Autodesk Fusion 360 part; units mm, degrees
(part 3 of 3)
extrude "Extruir4" cut sketch "Boceto5" against normal blind 3 contours S7 L81 L82 L83 L84 L85 L86 L87 L88 L89 L90 L91 L92 S8 L93 L94 L95 L96 L97 L98 L99 L100 L101 L102 L103 L104 L105 L106 L107 L108 L109 L110 L111 L112 L113 L114 L115 L116 L117 L118 L119 L120 L121 L122 L123 L124 S9 S10 L125 L126 | S15 L179 L180 S16 L181 L182 L183 L184 L185 L186 L187 L188 L189 L190 L191 L192 L193 L194 L195 L196 S17 L197 L198 L199 L200 L201 L202 L203 L204 S18 S19 L205 L206 L207 L208 S20 L209 L210 L211 L212 L213 L214 S21 L215 L216 L217 L218 S22 L219 L220 L221 L222 | L269 L270 S29 L271 L272 L273 L274 L275 L276 L277 L278 L279 L280 S30 L281 L282 S31 L283 L284 S32 L285 L286 L287 L288 L289 L290 L291 L292 L293 L294 L295 L296 L297 L298 L299 L300 L301 L302 L303 L304 L305 L306 L307 L308 S33 L309 L310 L311 L312 | L363 L364 S41 L365 L366 S42 L367 L368 L369 L370 L371 L372 S43 L373 L374 L375 L376 S44 L377 L378 L379 L380 L381 L382 L383 L384 S45 L385 L386 L387 L388 L389 L390 L391 L392 S46 L393 L394 L395 L396 L397 L398 L399 L400 L401 L402 L403 L404 L405 L406 L407 L408 L409 L410 | L451 L452 L453 L454 L455 L456 S57 L457 L458 L459 L460 L461 L462 L463 L464 L465 L466 S58 S59 S60 L467 L468 L469 L470 L471 L472 L473 L474 S61 L475 L476 L477 L478 L479 L480 L481 L482 L483 L484 L485 L486 L487 L488 S62 S63 S64 L489 L490 L491 L492 S65 | L541 L542 S70 L543 L544 L545 L546 L547 L548 L549 L550 L551 L552 L553 L554 L555 L556 S71 L557 L558 L559 L560 L561 L562 L563 L564 L565 L566 L567 L568 L569 L570 S72 L571 L572 L573 L574 L575 L576 L577 L578 L579 L580 L581 L582 L583 L584 S73 L585 L586 L587 L588 | L627 L628 L629 L630 L631 L632 L633 L634 L635 L636 L637 L638 L639 L640 L641 L642 L643 L644 L645 L646 L647 L648 L649 L650 L651 L652 L653 L654 L655 L656 L657 L658 L659 L660 L661 L662 L663 L664 L665 L666 L667 L668 L669 L670 L671 L672 L673 L674 L675 L676 S81 L677 L678 L679 L680 L681 L682 | S89 L723 L724 L725 L726 L727 L728 S90 L729 L730 L731 L732 L733 L734 S91 S92 S93 L735 L736 L737 L738 L739 L740 L741 L742 L743 L744 L745 L746 L747 L748 L749 L750 L751 L752 L753 L754 L755 L756 L757 L758 S94 S95 L759 L760 L761 L762 L763 L764 L765 L766 | S102 L815 L816 L817 L818 S103 L819 L820 L821 L822 L823 L824 L825 L826 L827 L828 L829 L830 L831 L832 L833 L834 L835 L836 S104 L837 L838 L839 L840 S105 L841 L842 S106 L843 L844 S107 L845 L846 L847 L848 L849 L850 S108 L851 L852 L853 L854 S109 L855 L856 | L903 L904 S117 L905 L906 S118 L907 L908 L909 L910 L911 L912 L913 L914 L915 L916 S119 L917 L918 L919 L920 L921 L922 L923 L924 L925 L926 L927 L928 L929 L930 L931 L932 L933 L934 S120 L935 L936 L937 L938 L939 L940 S121 L941 L942 L943 L944 | L985 L986 S129 S130 L987 L988 L989 L990 L991 L992 L993 L994 L995 L996 L997 L998 L999 L1000 L1001 L1002 S131 L1003 L1004 L1005 L1006 L1007 L1008 L1009 L1010 S132 L1011 L1012 L1013 L1014 L1015 L1016 L1017 L1018 L1019 L1020 L1021 L1022 S133 L1023 L1024 L1025 L1026 L1027 L1028 L1029 L1030 L1031 L1032 L1033 L1034 | S141 L1079 L1080 L1081 L1082 L1083 L1084 L1085 L1086 L1087 L1088 L1089 L1090 L1091 L1092 L1093 L1094 S142 L1095 L1096 L1097 L1098 S143 L1099 L1100 L1101 L1102 L1103 L1104 L1105 L1106 L1107 L1108 L1109 L1110 S144 L1111 L1112 L1113 L1114 S145 L1115 L1116 L1117 L1118 S146 L1119 L1120 L1121 L1122 L1123 L1124 L1125 L1126 bodies 2
sketch "Boceto7" plane through (0, -37, 0) normal (0, 1, 0) x (-1, 0, 0)
  line L0 (14.5856, 106.9791) -> (14.4281, 107.0187)
  line L1 (14.4281, 107.0187) -> (14.3014, 107.078)
  spline S0 degree 3 poles (14.3014, 107.078) (14.2318, 107.1106) (11.7179, 108.5531) (8.7151, 110.2835) knots 0 0 0 0 1 1 1 1
  line L2 (8.7151, 110.2835) -> (3.2554, 113.4298)
  line L3 (3.2554, 113.4298) -> (3.1368, 113.5206)
  spline S1 degree 3 poles (3.1368, 113.5206) (3.0715, 113.5705) (2.9644, 113.6706) (2.8986, 113.743) knots 0 0 0 0 1 1 1 1
  line L4 (2.8986, 113.743) -> (2.7791, 113.8747)
  line L5 (2.7791, 113.8747) -> (2.6095, 114.1591)
  line L6 (2.6095, 114.1591) -> (2.5502, 114.3319)
  line L7 (2.5502, 114.3319) -> (2.4909, 114.5047)
  line L8 (2.4909, 114.5047) -> (2.469, 114.6412)
  spline S2 degree 3 poles (2.469, 114.6412) (2.4006, 115.0677) (2.504, 115.4998) (2.7672, 115.888) knots 0 0 0 0 1 1 1 1
  line L9 (2.7672, 115.888) -> (2.8507, 116.0112)
  line L10 (2.8507, 116.0112) -> (2.9755, 116.136)
  line L11 (2.9755, 116.136) -> (3.1003, 116.2607)
  line L12 (3.1003, 116.2607) -> (3.2424, 116.3527)
  spline S3 degree 3 poles (3.2424, 116.3527) (3.3206, 116.4033) (3.4405, 116.4695) (3.509, 116.4999) knots 0 0 0 0 1 1 1 1
  line L13 (3.509, 116.4999) -> (3.6334, 116.5552)
  line L14 (3.6334, 116.5552) -> (3.9904, 116.6432)
  line L15 (3.9904, 116.6432) -> (4.2109, 116.6419)
  line L16 (4.2109, 116.6419) -> (4.4315, 116.6407)
  line L17 (4.4315, 116.6407) -> (4.5995, 116.5962)
  line L18 (4.5995, 116.5962) -> (4.7675, 116.5517)
  line L19 (4.7675, 116.5517) -> (4.9145, 116.4817)
  spline S4 degree 3 poles (4.9145, 116.4817) (5.0975, 116.3946) (15.7827, 110.2419) (15.9754, 110.1127) knots 0 0 0 0 1 1 1 1
  line L20 (15.9754, 110.1127) -> (16.1156, 110.0186)
  line L21 (16.1156, 110.0186) -> (16.2617, 109.8648)
  line L22 (16.2617, 109.8648) -> (16.4079, 109.7109)
  line L23 (16.4079, 109.7109) -> (16.497, 109.561)
  line L24 (16.497, 109.561) -> (16.586, 109.4111)
  line L25 (16.586, 109.4111) -> (16.7046, 109.0654)
  line L26 (16.7046, 109.0654) -> (16.7265, 108.9289)
  spline S5 degree 3 poles (16.7265, 108.9289) (16.7385, 108.8538) (16.7485, 108.7329) (16.7486, 108.6602) knots 0 0 0 0 1 1 1 1
  line L27 (16.7486, 108.6602) -> (16.7487, 108.5281)
  line L28 (16.7487, 108.5281) -> (16.7154, 108.3662)
  line L29 (16.7154, 108.3662) -> (16.682, 108.2044)
  line L30 (16.682, 108.2044) -> (16.6212, 108.0463)
  line L31 (16.6212, 108.0463) -> (16.5603, 107.8883)
  line L32 (16.5603, 107.8883) -> (16.4558, 107.7291)
  line L33 (16.4558, 107.7291) -> (16.3513, 107.5699)
  line L34 (16.3513, 107.5699) -> (16.1738, 107.4019)
  line L35 (16.1738, 107.4019) -> (15.9964, 107.234)
  line L36 (15.9964, 107.234) -> (15.6251, 107.0427)
  line L37 (15.6251, 107.0427) -> (15.4744, 106.9972)
  line L38 (15.4744, 106.9972) -> (15.3236, 106.9516)
  line L39 (15.3236, 106.9516) -> (15.1804, 106.9351)
  line L40 (15.1804, 106.9351) -> (15.0371, 106.9187)
  line L41 (15.0371, 106.9187) -> (14.8901, 106.9291)
  line L42 (14.8901, 106.9291) -> (14.7431, 106.9395)
  line L43 (14.7431, 106.9395) -> (14.5856, 106.9791)
  line L44 (-15.008, 106.9658) -> (-15.1472, 106.9935)
  line L45 (-15.1472, 106.9935) -> (-15.3104, 107.0614)
  line L46 (-15.3104, 107.0614) -> (-15.4735, 107.1293)
  line L47 (-15.4735, 107.1293) -> (-15.6249, 107.2305)
  line L48 (-15.6249, 107.2305) -> (-15.7763, 107.3318)
  line L49 (-15.7763, 107.3318) -> (-15.9106, 107.4743)
  spline S6 degree 3 poles (-15.9106, 107.4743) (-15.9844, 107.5526) (-16.0816, 107.6722) (-16.1266, 107.7401) knots 0 0 0 0 1 1 1 1
  line L50 (-16.1266, 107.7401) -> (-16.2083, 107.8634)
  line L51 (-16.2083, 107.8634) -> (-16.278, 108.0344)
  line L52 (-16.278, 108.0344) -> (-16.3477, 108.2054)
  line L53 (-16.3477, 108.2054) -> (-16.3823, 108.4044)
  line L54 (-16.3823, 108.4044) -> (-16.4168, 108.6034)
  line L55 (-16.4168, 108.6034) -> (-16.4028, 108.7786)
  line L56 (-16.4028, 108.7786) -> (-16.3888, 108.9539)
  line L57 (-16.3888, 108.9539) -> (-16.3374, 109.1312)
  line L58 (-16.3374, 109.1312) -> (-16.2861, 109.3085)
  line L59 (-16.2861, 109.3085) -> (-16.2151, 109.4495)
  spline S7 degree 3 poles (-16.2151, 109.4495) (-16.086, 109.7058) (-15.8768, 109.9466) (-15.6462, 110.1044) knots 0 0 0 0 1 1 1 1
  spline S8 degree 3 poles (-15.6462, 110.1044) (-15.4992, 110.205) (-4.6465, 116.4518) (-4.5256, 116.5054) knots 0 0 0 0 1 1 1 1
  spline S9 degree 3 poles (-4.5256, 116.5054) (-4.4621, 116.5336) (-4.3392, 116.5755) (-4.2526, 116.5985) knots 0 0 0 0 1 1 1 1
  line L60 (-4.2526, 116.5985) -> (-4.0951, 116.6404)
  line L61 (-4.0951, 116.6404) -> (-3.6121, 116.6404)
  line L62 (-3.6121, 116.6404) -> (-3.2783, 116.552)
  line L63 (-3.2783, 116.552) -> (-3.1092, 116.47)
  line L64 (-3.1092, 116.47) -> (-2.94, 116.3879)
  line L65 (-2.94, 116.3879) -> (-2.8017, 116.2831)
  spline S10 degree 3 poles (-2.8017, 116.2831) (-2.6357, 116.1572) (-2.5152, 116.0251) (-2.3869, 115.8283) knots 0 0 0 0 1 1 1 1
  line L66 (-2.3869, 115.8283) -> (-2.2913, 115.6818)
  line L67 (-2.2913, 115.6818) -> (-2.2308, 115.526)
  line L68 (-2.2308, 115.526) -> (-2.1703, 115.3701)
  line L69 (-2.1703, 115.3701) -> (-2.1404, 115.2138)
  line L70 (-2.1404, 115.2138) -> (-2.1105, 115.0576)
  line L71 (-2.1105, 115.0576) -> (-2.1105, 114.7235)
  line L72 (-2.1105, 114.7235) -> (-2.1437, 114.5616)
  line L73 (-2.1437, 114.5616) -> (-2.177, 114.3997)
  line L74 (-2.177, 114.3997) -> (-2.2405, 114.2466)
  line L75 (-2.2405, 114.2466) -> (-2.3041, 114.0935)
  line L76 (-2.3041, 114.0935) -> (-2.4037, 113.9421)
  line L77 (-2.4037, 113.9421) -> (-2.5034, 113.7907)
  line L78 (-2.5034, 113.7907) -> (-2.6482, 113.6524)
  spline S11 degree 3 poles (-2.6482, 113.6524) (-2.7278, 113.5763) (-2.845, 113.4803) (-2.9085, 113.4391) knots 0 0 0 0 1 1 1 1
  spline S12 degree 3 poles (-2.9085, 113.4391) (-3.069, 113.3348) (-13.7648, 107.1737) (-13.9105, 107.1015) knots 0 0 0 0 1 1 1 1
  spline S13 degree 3 poles (-13.9105, 107.1015) (-13.9755, 107.0693) (-14.0965, 107.0224) (-14.1795, 106.9973) knots 0 0 0 0 1 1 1 1
  line L79 (-14.1795, 106.9973) -> (-14.3302, 106.9516)
  line L80 (-14.3302, 106.9516) -> (-14.4735, 106.9354)
  line L81 (-14.4735, 106.9354) -> (-14.6167, 106.9192)
  line L82 (-14.6167, 106.9192) -> (-14.7427, 106.9287)
  spline S14 degree 3 poles (-14.7427, 106.9287) (-14.812, 106.9339) (-14.9314, 106.9506) (-15.008, 106.9658) knots 0 0 0 0 1 1 1 1
  line L83 (-0.2165, 120.1648) -> (-0.3912, 120.2066)
  line L84 (-0.3912, 120.2066) -> (-0.5457, 120.278)
  spline S15 degree 3 poles (-0.5457, 120.278) (-0.7389, 120.3673) (-0.8685, 120.4553) (-1.0261, 120.6045) knots 0 0 0 0 1 1 1 1
  line L85 (-1.0261, 120.6045) -> (-1.1493, 120.7211)
  line L86 (-1.1493, 120.7211) -> (-1.2389, 120.8471)
  spline S16 degree 3 poles (-1.2389, 120.8471) (-1.3602, 121.0178) (-1.4477, 121.1975) (-1.517, 121.4184) knots 0 0 0 0 1 1 1 1
  line L87 (-1.517, 121.4184) -> (-1.5749, 121.6032)
  line L88 (-1.5749, 121.6032) -> (-1.5749, 134.561)
  line L89 (-1.5749, 134.561) -> (-1.4807, 134.9143)
  line L90 (-1.4807, 134.9143) -> (-1.3974, 135.0842)
  line L91 (-1.3974, 135.0842) -> (-1.3141, 135.254)
  line L92 (-1.3141, 135.254) -> (-1.0954, 135.5423)
  line L93 (-1.0954, 135.5423) -> (-0.9572, 135.6569)
  spline S17 degree 3 poles (-0.9572, 135.6569) (-0.7085, 135.863) (-0.4228, 135.9976) (-0.1153, 136.0535) knots 0 0 0 0 1 1 1 1
  line L94 (-0.1153, 136.0535) -> (0.0422, 136.0821)
  line L95 (0.0422, 136.0821) -> (0.3152, 136.0831)
  line L96 (0.3152, 136.0831) -> (0.5147, 136.0422)
  line L97 (0.5147, 136.0422) -> (0.7142, 136.0013)
  line L98 (0.7142, 136.0013) -> (0.9242, 135.8966)
  line L99 (0.9242, 135.8966) -> (1.1342, 135.7918)
  line L100 (1.1342, 135.7918) -> (1.2665, 135.684)
  line L101 (1.2665, 135.684) -> (1.3987, 135.5761)
  line L102 (1.3987, 135.5761) -> (1.5149, 135.4361)
  line L103 (1.5149, 135.4361) -> (1.6311, 135.2961)
  line L104 (1.6311, 135.2961) -> (1.7356, 135.0832)
  line L105 (1.7356, 135.0832) -> (1.8401, 134.8704)
  line L106 (1.8401, 134.8704) -> (1.9212, 134.477)
  line L107 (1.9212, 134.477) -> (1.9216, 121.7502)
  line L108 (1.9216, 121.7502) -> (1.8994, 121.6137)
  spline S18 degree 3 poles (1.8994, 121.6137) (1.8873, 121.5386) (1.8538, 121.4063) (1.8249, 121.3197) knots 0 0 0 0 1 1 1 1
  line L109 (1.8249, 121.3197) -> (1.7725, 121.1622)
  line L110 (1.7725, 121.1622) -> (1.6845, 121.0047)
  line L111 (1.6845, 121.0047) -> (1.5964, 120.8472)
  line L112 (1.5964, 120.8472) -> (1.3968, 120.6454)
  line L113 (1.3968, 120.6454) -> (1.1973, 120.4437)
  line L114 (1.1973, 120.4437) -> (1.0515, 120.3631)
  spline S19 degree 3 poles (1.0515, 120.3631) (0.8617, 120.2581) (0.688, 120.1888) (0.5281, 120.154) knots 0 0 0 0 1 1 1 1
  line L115 (0.5281, 120.154) -> (0.3993, 120.126)
  line L116 (0.3993, 120.126) -> (0.1788, 120.1244)
  line L117 (0.1788, 120.1244) -> (-0.0417, 120.1229)
  line L118 (-0.0417, 120.1229) -> (-0.2165, 120.1648)
  spline S20 degree 3 poles (-14.9801, 128.7007) (-15.0601, 128.7176) (-15.1906, 128.7558) (-15.2699, 128.7857) knots 0 0 0 0 1 1 1 1
  line L119 (-15.2699, 128.7857) -> (-15.4143, 128.84)
  line L120 (-15.4143, 128.84) -> (-15.568, 128.9358)
  line L121 (-15.568, 128.9358) -> (-15.7218, 129.0317)
  line L122 (-15.7218, 129.0317) -> (-15.8482, 129.1487)
  line L123 (-15.8482, 129.1487) -> (-15.9746, 129.2657)
  line L124 (-15.9746, 129.2657) -> (-16.0679, 129.3965)
  line L125 (-16.0679, 129.3965) -> (-16.1612, 129.5272)
  line L126 (-16.1612, 129.5272) -> (-16.2425, 129.7025)
  line L127 (-16.2425, 129.7025) -> (-16.3237, 129.8777)
  line L128 (-16.3237, 129.8777) -> (-16.3619, 130.0247)
  line L129 (-16.3619, 130.0247) -> (-16.4001, 130.1717)
  line L130 (-16.4001, 130.1717) -> (-16.3965, 130.6757)
  line L131 (-16.3965, 130.6757) -> (-16.3412, 130.8605)
  line L132 (-16.3412, 130.8605) -> (-16.286, 131.0452)
  line L133 (-16.286, 131.0452) -> (-16.2207, 131.1755)
  spline S21 degree 3 poles (-16.2207, 131.1755) (-16.1848, 131.2471) (-16.1143, 131.3637) (-16.0641, 131.4345) knots 0 0 0 0 1 1 1 1
  line L134 (-16.0641, 131.4345) -> (-15.9729, 131.5632)
  line L135 (-15.9729, 131.5632) -> (-15.8303, 131.6939)
  line L136 (-15.8303, 131.6939) -> (-15.6878, 131.8247)
  line L137 (-15.6878, 131.8247) -> (-15.5198, 131.9239)
  spline S22 degree 3 poles (-15.5198, 131.9239) (-15.4274, 131.9784) (-12.9324, 133.421) (-9.9754, 135.1296) knots 0 0 0 0 1 1 1 1
  line L138 (-9.9754, 135.1296) -> (-4.5991, 138.2362)
  line L139 (-4.5991, 138.2362) -> (-4.1791, 138.3825)
  line L140 (-4.1791, 138.3825) -> (-3.57, 138.3832)
  line L141 (-3.57, 138.3832) -> (-3.4335, 138.3467)
  line L142 (-3.4335, 138.3467) -> (-3.297, 138.3101)
  line L143 (-3.297, 138.3101) -> (-3.0765, 138.2007)
  line L144 (-3.0765, 138.2007) -> (-2.856, 138.0912)
  line L145 (-2.856, 138.0912) -> (-2.646, 137.8802)
  line L146 (-2.646, 137.8802) -> (-2.436, 137.6691)
  line L147 (-2.436, 137.6691) -> (-2.3655, 137.549)
  spline S23 degree 3 poles (-2.3655, 137.549) (-2.2813, 137.4053) (-2.2082, 137.2289) (-2.1624, 137.0588) knots 0 0 0 0 1 1 1 1
  line L148 (-2.1624, 137.0588) -> (-2.1289, 136.9341)
  line L149 (-2.1289, 136.9341) -> (-2.1169, 136.7338)
  line L150 (-2.1169, 136.7338) -> (-2.1048, 136.5335)
  line L151 (-2.1048, 136.5335) -> (-2.1403, 136.3584)
  spline S24 degree 3 poles (-2.1403, 136.3584) (-2.1858, 136.1342) (-2.2581, 135.9423) (-2.3658, 135.7608) knots 0 0 0 0 1 1 1 1
  line L152 (-2.3658, 135.7608) -> (-2.4513, 135.6166)
  line L153 (-2.4513, 135.6166) -> (-2.5974, 135.4627)
  line L154 (-2.5974, 135.4627) -> (-2.7436, 135.3088)
  line L155 (-2.7436, 135.3088) -> (-2.8838, 135.2147)
  spline S25 degree 3 poles (-2.8838, 135.2147) (-2.9609, 135.163) (-5.4575, 133.7148) (-8.4318, 131.9965) knots 0 0 0 0 1 1 1 1
  line L156 (-8.4318, 131.9965) -> (-13.8397, 128.8724)
  line L157 (-13.8397, 128.8724) -> (-13.9972, 128.804)
  line L158 (-13.9972, 128.804) -> (-14.1547, 128.7357)
  line L159 (-14.1547, 128.7357) -> (-14.3017, 128.7046)
  line L160 (-14.3017, 128.7046) -> (-14.4487, 128.6735)
  line L161 (-14.4487, 128.6735) -> (-14.8345, 128.6701)
  line L162 (-14.8345, 128.6701) -> (-14.9801, 128.7007)
  spline S26 degree 3 poles (-4.2618, 96.0858) (-4.3304, 96.1044) (-4.4401, 96.1413) (-4.5056, 96.1677) knots 0 0 0 0 1 1 1 1
  line L163 (-4.5056, 96.1677) -> (-4.6247, 96.2158)
  line L164 (-4.6247, 96.2158) -> (-10.0722, 99.3629)
  spline S27 degree 3 poles (-10.0722, 99.3629) (-13.0684, 101.0939) (-15.5752, 102.5473) (-15.643, 102.5927) knots 0 0 0 0 1 1 1 1
  line L165 (-15.643, 102.5927) -> (-15.7662, 102.6754)
  line L166 (-15.7662, 102.6754) -> (-16.0158, 102.925)
  line L167 (-16.0158, 102.925) -> (-16.1184, 103.0821)
  line L168 (-16.1184, 103.0821) -> (-16.2209, 103.2393)
  line L169 (-16.2209, 103.2393) -> (-16.2849, 103.4052)
  line L170 (-16.2849, 103.4052) -> (-16.3489, 103.5711)
  line L171 (-16.3489, 103.5711) -> (-16.3829, 103.7666)
  line L172 (-16.3829, 103.7666) -> (-16.4168, 103.9621)
  line L173 (-16.4168, 103.9621) -> (-16.4028, 104.1373)
  line L174 (-16.4028, 104.1373) -> (-16.3888, 104.3126)
  line L175 (-16.3888, 104.3126) -> (-16.3363, 104.4943)
  line L176 (-16.3363, 104.4943) -> (-16.2839, 104.6761)
  line L177 (-16.2839, 104.6761) -> (-16.1995, 104.8328)
  line L178 (-16.1995, 104.8328) -> (-16.1152, 104.9895)
  line L179 (-16.1152, 104.9895) -> (-16.0086, 105.121)
  spline S28 degree 3 poles (-16.0086, 105.121) (-15.8856, 105.2726) (-15.7612, 105.3819) (-15.5741, 105.5029) knots 0 0 0 0 1 1 1 1
  line L180 (-15.5741, 105.5029) -> (-15.4418, 105.5883)
  line L181 (-15.4418, 105.5883) -> (-15.2773, 105.6518)
  line L182 (-15.2773, 105.6518) -> (-15.1127, 105.7153)
  line L183 (-15.1127, 105.7153) -> (-14.9172, 105.7492)
  line L184 (-14.9172, 105.7492) -> (-14.7217, 105.7832)
  line L185 (-14.7217, 105.7832) -> (-14.5465, 105.7692)
  line L186 (-14.5465, 105.7692) -> (-14.3712, 105.7552)
  line L187 (-14.3712, 105.7552) -> (-14.1932, 105.7036)
  spline S29 degree 3 poles (-14.1932, 105.7036) (-14.0953, 105.6752) (-13.9757, 105.632) (-13.9274, 105.6075) knots 0 0 0 0 1 1 1 1
  spline S30 degree 3 poles (-13.9274, 105.6075) (-13.7892, 105.5374) (-3.0607, 99.3373) (-2.9105, 99.2406) knots 0 0 0 0 1 1 1 1
  line L188 (-2.9105, 99.2406) -> (-2.776, 99.1541)
  line L189 (-2.776, 99.1541) -> (-2.6464, 99.0264)
  line L190 (-2.6464, 99.0264) -> (-2.5167, 98.8986)
  line L191 (-2.5167, 98.8986) -> (-2.432, 98.7737)
  spline S31 degree 3 poles (-2.432, 98.7737) (-2.3086, 98.5917) (-2.2438, 98.4542) (-2.1837, 98.2468) knots 0 0 0 0 1 1 1 1
  line L192 (-2.1837, 98.2468) -> (-2.1304, 98.0629)
  line L193 (-2.1304, 98.0629) -> (-2.1176, 97.8832)
  line L194 (-2.1176, 97.8832) -> (-2.1049, 97.7036)
  line L195 (-2.1049, 97.7036) -> (-2.1576, 97.3887)
  line L196 (-2.1576, 97.3887) -> (-2.2132, 97.2312)
  spline S32 degree 3 poles (-2.2132, 97.2312) (-2.2806, 97.0402) (-2.3908, 96.8417) (-2.5188, 96.6805) knots 0 0 0 0 1 1 1 1
  line L197 (-2.5188, 96.6805) -> (-2.6142, 96.5603)
  line L198 (-2.6142, 96.5603) -> (-2.7542, 96.4448)
  line L199 (-2.7542, 96.4448) -> (-2.8943, 96.3293)
  line L200 (-2.8943, 96.3293) -> (-3.0536, 96.2468)
  spline S33 degree 3 poles (-3.0536, 96.2468) (-3.2371, 96.152) (-3.3668, 96.1052) (-3.5595, 96.0642) knots 0 0 0 0 1 1 1 1
  line L201 (-3.5595, 96.0642) -> (-3.696, 96.0353)
  line L202 (-3.696, 96.0353) -> (-3.9166, 96.0436)
  line L203 (-3.9166, 96.0436) -> (-4.1371, 96.052)
  line L204 (-4.1371, 96.052) -> (-4.2618, 96.0858)
  line L205 (18.4918, 109.3246) -> (18.2923, 109.3899)
  line L206 (18.2923, 109.3899) -> (18.1589, 109.4691)
  spline S34 degree 3 poles (18.1589, 109.4691) (18.0854, 109.5126) (17.9724, 109.591) (17.9076, 109.6432) knots 0 0 0 0 1 1 1 1
  line L207 (17.9076, 109.6432) -> (17.7897, 109.7381)
  line L208 (17.7897, 109.7381) -> (17.6666, 109.8847)
  line L209 (17.6666, 109.8847) -> (17.5434, 110.0314)
  line L210 (17.5434, 110.0314) -> (17.4504, 110.2204)
  line L211 (17.4504, 110.2204) -> (17.3573, 110.4095)
  line L212 (17.3573, 110.4095) -> (17.2632, 110.7455)
  line L213 (17.2632, 110.7455) -> (17.2508, 123.4303)
  line L214 (17.2508, 123.4303) -> (17.2729, 123.6239)
  line L215 (17.2729, 123.6239) -> (17.295, 123.8175)
  line L216 (17.295, 123.8175) -> (17.3548, 123.9956)
  line L217 (17.3548, 123.9956) -> (17.4147, 124.1736)
  line L218 (17.4147, 124.1736) -> (17.5002, 124.3165)
  spline S35 degree 3 poles (17.5002, 124.3165) (17.5472, 124.3951) (17.632, 124.5138) (17.6887, 124.5803) knots 0 0 0 0 1 1 1 1
  line L219 (17.6887, 124.5803) -> (17.7918, 124.7012)
  line L220 (17.7918, 124.7012) -> (17.937, 124.8179)
  line L221 (17.937, 124.8179) -> (18.0823, 124.9345)
  line L222 (18.0823, 124.9345) -> (18.2503, 125.0161)
  line L223 (18.2503, 125.0161) -> (18.4183, 125.0977)
  line L224 (18.4183, 125.0977) -> (18.7543, 125.1929)
  line L225 (18.7543, 125.1929) -> (19.2794, 125.1926)
  line L226 (19.2794, 125.1926) -> (19.4523, 125.1441)
  line L227 (19.4523, 125.1441) -> (19.6252, 125.0955)
  line L228 (19.6252, 125.0955) -> (19.9422, 124.9334)
  line L229 (19.9422, 124.9334) -> (20.0636, 124.8399)
  spline S36 degree 3 poles (20.0636, 124.8399) (20.1304, 124.7885) (20.2391, 124.6881) (20.305, 124.6169) knots 0 0 0 0 1 1 1 1
  line L230 (20.305, 124.6169) -> (20.425, 124.4874)
  line L231 (20.425, 124.4874) -> (20.5195, 124.3263)
  line L232 (20.5195, 124.3263) -> (20.6139, 124.1653)
  line L233 (20.6139, 124.1653) -> (20.7495, 123.7663)
  line L234 (20.7495, 123.7663) -> (20.7495, 110.7035)
  line L235 (20.7495, 110.7035) -> (20.7021, 110.54)
  line L236 (20.7021, 110.54) -> (20.6547, 110.3765)
  line L237 (20.6547, 110.3765) -> (20.5725, 110.2131)
  line L238 (20.5725, 110.2131) -> (20.4904, 110.0497)
  line L239 (20.4904, 110.0497) -> (20.373, 109.9023)
  line L240 (20.373, 109.9023) -> (20.2556, 109.755)
  line L241 (20.2556, 109.755) -> (20.1245, 109.6488)
  spline S37 degree 3 poles (20.1245, 109.6488) (19.8952, 109.4632) (19.6372, 109.3357) (19.3653, 109.2738) knots 0 0 0 0 1 1 1 1
  line L242 (19.3653, 109.2738) -> (19.2374, 109.2446)
  line L243 (19.2374, 109.2446) -> (18.9643, 109.252)
  line L244 (18.9643, 109.252) -> (18.6913, 109.2594)
  line L245 (18.6913, 109.2594) -> (18.4918, 109.3246)
  spline S38 degree 3 poles (3.947, 96.0562) (3.6813, 96.1032) (3.4436, 96.2003) (3.2159, 96.3547) knots 0 0 0 0 1 1 1 1
  line L246 (3.2159, 96.3547) -> (3.0924, 96.4384)
  line L247 (3.0924, 96.4384) -> (2.8386, 96.6956)
  line L248 (2.8386, 96.6956) -> (2.7384, 96.8488)
  line L249 (2.7384, 96.8488) -> (2.6382, 97.0019)
  line L250 (2.6382, 97.0019) -> (2.5742, 97.1678)
  line L251 (2.5742, 97.1678) -> (2.5102, 97.3337)
  line L252 (2.5102, 97.3337) -> (2.4764, 97.5292)
  line L253 (2.4764, 97.5292) -> (2.4425, 97.7247)
  line L254 (2.4425, 97.7247) -> (2.4711, 98.0549)
  line L255 (2.4711, 98.0549) -> (2.5105, 98.2052)
  spline S39 degree 3 poles (2.5105, 98.2052) (2.6122, 98.5936) (2.8445, 98.9405) (3.1621, 99.1785) knots 0 0 0 0 1 1 1 1
  line L256 (3.1621, 99.1785) -> (3.2764, 99.2641)
  line L257 (3.2764, 99.2641) -> (8.7367, 102.4202)
  line L258 (8.7367, 102.4202) -> (14.1971, 105.5763)
  line L259 (14.1971, 105.5763) -> (14.5336, 105.714)
  line L260 (14.5336, 105.714) -> (14.9321, 105.7832)
  line L261 (14.9321, 105.7832) -> (15.1074, 105.7692)
  line L262 (15.1074, 105.7692) -> (15.2826, 105.7552)
  line L263 (15.2826, 105.7552) -> (15.6461, 105.6499)
  line L264 (15.6461, 105.6499) -> (15.9623, 105.4816)
  line L265 (15.9623, 105.4816) -> (16.0977, 105.3723)
  line L266 (16.0977, 105.3723) -> (16.2331, 105.2631)
  line L267 (16.2331, 105.2631) -> (16.3447, 105.1271)
  line L268 (16.3447, 105.1271) -> (16.4563, 104.9911)
  line L269 (16.4563, 104.9911) -> (16.5586, 104.7811)
  line L270 (16.5586, 104.7811) -> (16.661, 104.5711)
  line L271 (16.661, 104.5711) -> (16.6955, 104.4346)
  line L272 (16.6955, 104.4346) -> (16.73, 104.2981)
  line L273 (16.73, 104.2981) -> (16.7415, 104.0986)
  line L274 (16.7415, 104.0986) -> (16.753, 103.8991)
  line L275 (16.753, 103.8991) -> (16.7101, 103.692)
  line L276 (16.7101, 103.692) -> (16.6671, 103.485)
  line L277 (16.6671, 103.485) -> (16.5626, 103.272)
  line L278 (16.5626, 103.272) -> (16.458, 103.059)
  line L279 (16.458, 103.059) -> (16.3418, 102.919)
  line L280 (16.3418, 102.919) -> (16.2256, 102.779)
  line L281 (16.2256, 102.779) -> (15.9743, 102.576)
  line L282 (15.9743, 102.576) -> (10.5599, 99.4468)
  spline S40 degree 3 poles (10.5599, 99.4468) (7.5821, 97.7257) (5.0794, 96.283) (4.9985, 96.2406) knots 0 0 0 0 1 1 1 1
  spline S41 degree 3 poles (4.9985, 96.2406) (4.7337, 96.102) (4.502, 96.0412) (4.22, 96.0365) knots 0 0 0 0 1 1 1 1
  line L283 (4.22, 96.0365) -> (4.0716, 96.0341)
  line L284 (4.0716, 96.0341) -> (3.947, 96.0562)
  line L285 (-19.0547, 109.2861) -> (-19.2294, 109.328)
  line L286 (-19.2294, 109.328) -> (-19.3873, 109.4009)
  line L287 (-19.3873, 109.4009) -> (-19.5453, 109.4739)
  line L288 (-19.5453, 109.4739) -> (-19.6752, 109.5666)
  line L289 (-19.6752, 109.5666) -> (-19.8051, 109.6593)
  line L290 (-19.8051, 109.6593) -> (-19.9444, 109.807)
  line L291 (-19.9444, 109.807) -> (-20.0838, 109.9547)
  line L292 (-20.0838, 109.9547) -> (-20.1723, 110.1038)
  line L293 (-20.1723, 110.1038) -> (-20.2609, 110.2528)
  line L294 (-20.2609, 110.2528) -> (-20.3203, 110.4257)
  line L295 (-20.3203, 110.4257) -> (-20.3798, 110.5985)
  line L296 (-20.3798, 110.5985) -> (-20.4022, 110.7455)
  line L297 (-20.4022, 110.7455) -> (-20.4246, 110.8925)
  line L298 (-20.4246, 110.8925) -> (-20.4129, 123.7243)
  line L299 (-20.4129, 123.7243) -> (-20.3744, 123.8608)
  line L300 (-20.3744, 123.8608) -> (-20.3359, 123.9973)
  line L301 (-20.3359, 123.9973) -> (-20.1329, 124.4173)
  line L302 (-20.1329, 124.4173) -> (-20.0167, 124.5574)
  line L303 (-20.0167, 124.5574) -> (-19.9005, 124.6974)
  line L304 (-19.9005, 124.6974) -> (-19.7683, 124.8055)
  line L305 (-19.7683, 124.8055) -> (-19.636, 124.9136)
  line L306 (-19.636, 124.9136) -> (-19.216, 125.1174)
  line L307 (-19.216, 125.1174) -> (-18.922, 125.1923)
  line L308 (-18.922, 125.1923) -> (-18.418, 125.1923)
  line L309 (-18.418, 125.1923) -> (-18.271, 125.155)
  line L310 (-18.271, 125.155) -> (-18.1239, 125.1177)
  line L311 (-18.1239, 125.1177) -> (-17.9139, 125.0144)
  line L312 (-17.9139, 125.0144) -> (-17.7039, 124.9111)
  line L313 (-17.7039, 124.9111) -> (-17.5551, 124.7873)
  line L314 (-17.5551, 124.7873) -> (-17.4062, 124.6635)
  line L315 (-17.4062, 124.6635) -> (-17.1881, 124.3753)
  line L316 (-17.1881, 124.3753) -> (-17.1045, 124.2073)
  line L317 (-17.1045, 124.2073) -> (-17.021, 124.0393)
  line L318 (-17.021, 124.0393) -> (-16.9739, 123.8608)
  line L319 (-16.9739, 123.8608) -> (-16.9269, 123.6823)
  line L320 (-16.9269, 123.6823) -> (-16.9269, 110.7455)
  line L321 (-16.9269, 110.7455) -> (-16.9659, 110.5985)
  line L322 (-16.9659, 110.5985) -> (-17.005, 110.4515)
  line L323 (-17.005, 110.4515) -> (-17.1675, 110.101)
  line L324 (-17.1675, 110.101) -> (-17.3525, 109.8424)
  line L325 (-17.3525, 109.8424) -> (-17.4757, 109.7258)
  spline S42 degree 3 poles (-17.4757, 109.7258) (-17.6334, 109.5765) (-17.7629, 109.4886) (-17.9568, 109.399) knots 0 0 0 0 1 1 1 1
  line L326 (-17.9568, 109.399) -> (-18.112, 109.3273)
  line L327 (-18.112, 109.3273) -> (-18.2755, 109.2871)
  line L328 (-18.2755, 109.2871) -> (-18.439, 109.2469)
  line L329 (-18.439, 109.2469) -> (-18.6595, 109.2456)
  line L330 (-18.6595, 109.2456) -> (-18.88, 109.2442)
  line L331 (-18.88, 109.2442) -> (-19.0547, 109.2861)
  line L332 (14.4687, 128.7571) -> (14.2573, 128.8298)
  line L333 (14.2573, 128.8298) -> (8.8089, 131.9757)
  spline S43 degree 3 poles (8.8089, 131.9757) (5.8122, 133.7059) (3.3084, 135.1553) (3.2449, 135.1966) knots 0 0 0 0 1 1 1 1
  spline S44 degree 3 poles (3.2449, 135.1966) (3.1814, 135.238) (3.0739, 135.3245) (3.0062, 135.3889) knots 0 0 0 0 1 1 1 1
  line L334 (3.0062, 135.3889) -> (2.8829, 135.506)
  line L335 (2.8829, 135.506) -> (2.7904, 135.6353)
  line L336 (2.7904, 135.6353) -> (2.698, 135.7646)
  line L337 (2.698, 135.7646) -> (2.6167, 135.9398)
  line L338 (2.6167, 135.9398) -> (2.5355, 136.1151)
  line L339 (2.5355, 136.1151) -> (2.4975, 136.2621)
  line L340 (2.4975, 136.2621) -> (2.4596, 136.4091)
  line L341 (2.4596, 136.4091) -> (2.4596, 136.8921)
  line L342 (2.4596, 136.8921) -> (2.5355, 137.1861)
  line L343 (2.5355, 137.1861) -> (2.6167, 137.3614)
  line L344 (2.6167, 137.3614) -> (2.698, 137.5366)
  line L345 (2.698, 137.5366) -> (2.7904, 137.6659)
  line L346 (2.7904, 137.6659) -> (2.8829, 137.7952)
  line L347 (2.8829, 137.7952) -> (3.0062, 137.9118)
  spline S45 degree 3 poles (3.0062, 137.9118) (3.1638, 138.0609) (3.2933, 138.149) (3.4866, 138.2383) knots 0 0 0 0 1 1 1 1
  line L348 (3.4866, 138.2383) -> (3.6411, 138.3097)
  line L349 (3.6411, 138.3097) -> (3.9904, 138.3934)
  line L350 (3.9904, 138.3934) -> (4.4105, 138.3934)
  line L351 (4.4105, 138.3934) -> (4.756, 138.3106)
  line L352 (4.756, 138.3106) -> (4.8877, 138.2508)
  spline S46 degree 3 poles (4.8877, 138.2508) (5.059, 138.173) (15.8375, 131.9473) (16.0037, 131.8301) knots 0 0 0 0 1 1 1 1
  line L353 (16.0037, 131.8301) -> (16.1302, 131.7409)
  line L354 (16.1302, 131.7409) -> (16.2696, 131.5932)
  line L355 (16.2696, 131.5932) -> (16.4089, 131.4455)
  line L356 (16.4089, 131.4455) -> (16.4975, 131.2965)
  line L357 (16.4975, 131.2965) -> (16.586, 131.1474)
  line L358 (16.586, 131.1474) -> (16.6455, 130.9746)
  line L359 (16.6455, 130.9746) -> (16.7049, 130.8017)
  line L360 (16.7049, 130.8017) -> (16.7294, 130.6442)
  line L361 (16.7294, 130.6442) -> (16.7539, 130.4867)
  line L362 (16.7539, 130.4867) -> (16.742, 130.3158)
  line L363 (16.742, 130.3158) -> (16.7301, 130.1449)
  line L364 (16.7301, 130.1449) -> (16.6955, 130.0114)
  spline S47 degree 3 poles (16.6955, 130.0114) (16.6465, 129.8223) (16.5698, 129.6488) (16.4605, 129.4797) knots 0 0 0 0 1 1 1 1
  line L365 (16.4605, 129.4797) -> (16.3661, 129.3337)
  line L366 (16.3661, 129.3337) -> (16.2372, 129.1994)
  line L367 (16.2372, 129.1994) -> (16.1082, 129.0652)
  line L368 (16.1082, 129.0652) -> (15.959, 128.9654)
  line L369 (15.959, 128.9654) -> (15.8099, 128.8656)
  line L370 (15.8099, 128.8656) -> (15.4991, 128.7364)
  line L371 (15.4991, 128.7364) -> (15.3521, 128.7036)
  line L372 (15.3521, 128.7036) -> (15.2051, 128.6709)
  line L373 (15.2051, 128.6709) -> (14.6801, 128.6844)
  line L374 (14.6801, 128.6844) -> (14.4687, 128.7571)
  spline S48 degree 3 poles (-4.151, 117.8211) (-4.2357, 117.8375) (-4.3676, 117.8737) (-4.4441, 117.9015) knots 0 0 0 0 1 1 1 1
  line L375 (-4.4441, 117.9015) -> (-4.5831, 117.9522)
  line L376 (-4.5831, 117.9522) -> (-10.083, 121.1192)
  line L377 (-10.083, 121.1192) -> (-15.5828, 124.2861)
  line L378 (-15.5828, 124.2861) -> (-15.6884, 124.3646)
  spline S49 degree 3 poles (-15.6884, 124.3646) (-15.7465, 124.4078) (-15.8441, 124.4941) (-15.9054, 124.5563) knots 0 0 0 0 1 1 1 1
  line L379 (-15.9054, 124.5563) -> (-16.0168, 124.6694)
  line L380 (-16.0168, 124.6694) -> (-16.1204, 124.8264)
  line L381 (-16.1204, 124.8264) -> (-16.2239, 124.9833)
  line L382 (-16.2239, 124.9833) -> (-16.3489, 125.3075)
  line L383 (-16.3489, 125.3075) -> (-16.3829, 125.5029)
  line L384 (-16.3829, 125.5029) -> (-16.4168, 125.6984)
  line L385 (-16.4168, 125.6984) -> (-16.4028, 125.8737)
  line L386 (-16.4028, 125.8737) -> (-16.3888, 126.0489)
  line L387 (-16.3888, 126.0489) -> (-16.3363, 126.2307)
  line L388 (-16.3363, 126.2307) -> (-16.2839, 126.4125)
  line L389 (-16.2839, 126.4125) -> (-16.1992, 126.57)
  line L390 (-16.1992, 126.57) -> (-16.1145, 126.7275)
  line L391 (-16.1145, 126.7275) -> (-15.8904, 127.0049)
  line L392 (-15.8904, 127.0049) -> (-15.6216, 127.2188)
  line L393 (-15.6216, 127.2188) -> (-15.4657, 127.3016)
  spline S50 degree 3 poles (-15.4657, 127.3016) (-15.2046, 127.4402) (-14.9145, 127.5149) (-14.6377, 127.5146) knots 0 0 0 0 1 1 1 1
  line L394 (-14.6377, 127.5146) -> (-14.5117, 127.5145)
  line L395 (-14.5117, 127.5145) -> (-14.3139, 127.4737)
  line L396 (-14.3139, 127.4737) -> (-14.1161, 127.4328)
  line L397 (-14.1161, 127.4328) -> (-13.9464, 127.3511)
  spline S51 degree 3 poles (-13.9464, 127.3511) (-13.853, 127.3062) (-11.3296, 125.8591) (-8.3388, 124.1353) knots 0 0 0 0 1 1 1 1
  line L398 (-8.3388, 124.1353) -> (-2.9009, 121.0012)
  line L399 (-2.9009, 121.0012) -> (-2.7814, 120.9093)
  spline S52 degree 3 poles (-2.7814, 120.9093) (-2.6252, 120.7891) (-2.4901, 120.6371) (-2.3742, 120.4511) knots 0 0 0 0 1 1 1 1
  line L400 (-2.3742, 120.4511) -> (-2.2803, 120.3006)
  line L401 (-2.2803, 120.3006) -> (-2.2286, 120.163)
  spline S53 degree 3 poles (-2.2286, 120.163) (-2.2001, 120.0873) (-2.1619, 119.9532) (-2.1436, 119.8649) knots 0 0 0 0 1 1 1 1
  line L402 (-2.1436, 119.8649) -> (-2.1105, 119.7043)
  line L403 (-2.1105, 119.7043) -> (-2.1105, 119.3648)
  line L404 (-2.1105, 119.3648) -> (-2.1437, 119.2029)
  line L405 (-2.1437, 119.2029) -> (-2.177, 119.041)
  line L406 (-2.177, 119.041) -> (-2.2399, 118.8894)
  spline S54 degree 3 poles (-2.2399, 118.8894) (-2.2745, 118.806) (-2.3408, 118.6784) (-2.3871, 118.6059) knots 0 0 0 0 1 1 1 1
  line L407 (-2.3871, 118.6059) -> (-2.4713, 118.474)
  line L408 (-2.4713, 118.474) -> (-2.751, 118.1867)
  line L409 (-2.751, 118.1867) -> (-2.8665, 118.1075)
  spline S55 degree 3 poles (-2.8665, 118.1075) (-3.1626, 117.9043) (-3.4886, 117.7988) (-3.836, 117.7938) knots 0 0 0 0 1 1 1 1
  line L410 (-3.836, 117.7938) -> (-3.9969, 117.7914)
  line L411 (-3.9969, 117.7914) -> (-4.151, 117.8211)
  line L412 (-0.2165, 98.4074) -> (-0.3912, 98.4493)
  line L413 (-0.3912, 98.4493) -> (-0.5457, 98.5207)
  spline S56 degree 3 poles (-0.5457, 98.5207) (-0.7389, 98.6099) (-0.8685, 98.698) (-1.0261, 98.8471) knots 0 0 0 0 1 1 1 1
  line L414 (-1.0261, 98.8471) -> (-1.1493, 98.9638)
  line L415 (-1.1493, 98.9638) -> (-1.3343, 99.2224)
  line L416 (-1.3343, 99.2224) -> (-1.4153, 99.3976)
  line L417 (-1.4153, 99.3976) -> (-1.4963, 99.5728)
  line L418 (-1.4963, 99.5728) -> (-1.5749, 99.8878)
  line L419 (-1.5749, 99.8878) -> (-1.5749, 112.7616)
  line L420 (-1.5749, 112.7616) -> (-1.5467, 112.8981)
  spline S57 degree 3 poles (-1.5467, 112.8981) (-1.5312, 112.9732) (-1.4908, 113.1069) (-1.4568, 113.1952) knots 0 0 0 0 1 1 1 1
  line L421 (-1.4568, 113.1952) -> (-1.3951, 113.3557)
  line L422 (-1.3951, 113.3557) -> (-1.3096, 113.488)
  spline S58 degree 3 poles (-1.3096, 113.488) (-1.1875, 113.6768) (-1.0688, 113.8118) (-0.9223, 113.9284) knots 0 0 0 0 1 1 1 1
  line L423 (-0.9223, 113.9284) -> (-0.7947, 114.03)
  line L424 (-0.7947, 114.03) -> (-0.6388, 114.1128)
  spline S59 degree 3 poles (-0.6388, 114.1128) (-0.3776, 114.2514) (-0.0876, 114.326) (0.1892, 114.3258) knots 0 0 0 0 1 1 1 1
  line L425 (0.1892, 114.3258) -> (0.3152, 114.3255)
  line L426 (0.3152, 114.3255) -> (0.5147, 114.2847)
  line L427 (0.5147, 114.2847) -> (0.7142, 114.2438)
  line L428 (0.7142, 114.2438) -> (0.9242, 114.139)
  line L429 (0.9242, 114.139) -> (1.1342, 114.0343)
  line L430 (1.1342, 114.0343) -> (1.2665, 113.9265)
  line L431 (1.2665, 113.9265) -> (1.3987, 113.8186)
  line L432 (1.3987, 113.8186) -> (1.6311, 113.5386)
  line L433 (1.6311, 113.5386) -> (1.7356, 113.3257)
  line L434 (1.7356, 113.3257) -> (1.8401, 113.1129)
  line L435 (1.8401, 113.1129) -> (1.8807, 112.9162)
  line L436 (1.8807, 112.9162) -> (1.9212, 112.7195)
  line L437 (1.9212, 112.7195) -> (1.9216, 99.9927)
  line L438 (1.9216, 99.9927) -> (1.8778, 99.7197)
  line L439 (1.8778, 99.7197) -> (1.7592, 99.374)
  line L440 (1.7592, 99.374) -> (1.5811, 99.0742)
  line L441 (1.5811, 99.0742) -> (1.2813, 98.7586)
  line L442 (1.2813, 98.7586) -> (1.1658, 98.6802)
  spline S60 degree 3 poles (1.1658, 98.6802) (0.9532, 98.536) (0.711, 98.4309) (0.4922, 98.3879) knots 0 0 0 0 1 1 1 1
  line L443 (0.4922, 98.3879) -> (0.3993, 98.3697)
  line L444 (0.3993, 98.3697) -> (0.1788, 98.3676)
  line L445 (0.1788, 98.3676) -> (-0.0417, 98.3654)
  line L446 (-0.0417, 98.3654) -> (-0.2165, 98.4074)
  spline S61 degree 3 poles (3.8806, 117.8246) (3.6716, 117.8678) (3.4777, 117.9415) (3.3069, 118.0427) knots 0 0 0 0 1 1 1 1
  line L447 (3.3069, 118.0427) -> (3.1695, 118.1242)
  line L448 (3.1695, 118.1242) -> (2.867, 118.4043)
  line L449 (2.867, 118.4043) -> (2.64, 118.747)
  line L450 (2.64, 118.747) -> (2.5873, 118.8731)
  spline S62 degree 3 poles (2.5873, 118.8731) (2.5584, 118.9424) (2.5191, 119.0592) (2.5001, 119.1327) knots 0 0 0 0 1 1 1 1
  line L451 (2.5001, 119.1327) -> (2.4655, 119.2663)
  line L452 (2.4655, 119.2663) -> (2.4531, 119.4414)
  line L453 (2.4531, 119.4414) -> (2.4407, 119.6165)
  line L454 (2.4407, 119.6165) -> (2.4666, 119.7766)
  line L455 (2.4666, 119.7766) -> (2.4924, 119.9366)
  line L456 (2.4924, 119.9366) -> (2.543, 120.0853)
  spline S63 degree 3 poles (2.543, 120.0853) (2.666, 120.4472) (2.9021, 120.7612) (3.2134, 120.9768) knots 0 0 0 0 1 1 1 1
  spline S64 degree 3 poles (3.2134, 120.9768) (3.2973, 121.035) (14.1137, 127.2678) (14.2431, 127.3327) knots 0 0 0 0 1 1 1 1
  spline S65 degree 3 poles (14.2431, 127.3327) (14.3718, 127.3971) (14.5821, 127.4647) (14.7417, 127.493) knots 0 0 0 0 1 1 1 1
  line L457 (14.7417, 127.493) -> (14.8663, 127.515)
  line L458 (14.8663, 127.515) -> (15.0042, 127.5148)
  line L459 (15.0042, 127.5148) -> (15.1421, 127.5145)
  line L460 (15.1421, 127.5145) -> (15.3388, 127.4739)
  line L461 (15.3388, 127.4739) -> (15.5355, 127.4333)
  line L462 (15.5355, 127.4333) -> (15.7483, 127.3288)
  line L463 (15.7483, 127.3288) -> (15.9612, 127.2242)
  line L464 (15.9612, 127.2242) -> (16.2117, 127.0208)
  line L465 (16.2117, 127.0208) -> (16.3352, 126.8742)
  line L466 (16.3352, 126.8742) -> (16.4587, 126.7275)
  line L467 (16.4587, 126.7275) -> (16.6624, 126.3075)
  line L468 (16.6624, 126.3075) -> (16.7357, 126.0344)
  line L469 (16.7357, 126.0344) -> (16.7373, 125.5094)
  line L470 (16.7373, 125.5094) -> (16.6987, 125.3624)
  line L471 (16.6987, 125.3624) -> (16.6601, 125.2154)
  line L472 (16.6601, 125.2154) -> (16.5778, 125.038)
  line L473 (16.5778, 125.038) -> (16.4955, 124.8605)
  line L474 (16.4955, 124.8605) -> (16.2661, 124.5557)
  line L475 (16.2661, 124.5557) -> (16.1449, 124.455)
  spline S66 degree 3 poles (16.1449, 124.455) (16.0783, 124.3997) (15.9766, 124.3246) (15.9189, 124.2882) knots 0 0 0 0 1 1 1 1
  spline S67 degree 3 poles (15.9189, 124.2882) (15.8613, 124.2519) (13.3806, 122.8204) (10.4063, 121.1072) knots 0 0 0 0 1 1 1 1
  line L476 (10.4063, 121.1072) -> (4.9985, 117.9923)
  line L477 (4.9985, 117.9923) -> (4.841, 117.9247)
  line L478 (4.841, 117.9247) -> (4.6835, 117.857)
  line L479 (4.6835, 117.857) -> (4.5365, 117.8259)
  line L480 (4.5365, 117.8259) -> (4.3895, 117.7949)
  line L481 (4.3895, 117.7949) -> (4.2153, 117.7931)
  line L482 (4.2153, 117.7931) -> (4.0412, 117.7914)
  line L483 (4.0412, 117.7914) -> (3.8806, 117.8246)
  line L484 (-43, 3) -> (-35.6412, 3)
  line L485 (-35.6412, 3) -> (-35.6412, 0)
  line L486 (-35.6412, 0) -> (-20.6412, 0)
  line L487 (-20.6412, 0) -> (-20.6412, 3)
  line L488 (-20.6412, 3) -> (-9.4275, 3)
  line L489 (-9.4275, 3) -> (-9.4275, 0)
  line L490 (-9.4275, 0) -> (5.5725, 0)
  line L491 (5.5725, 0) -> (5.5725, 3)
  line L492 (5.5725, 3) -> (16.7863, 3)
  line L493 (16.7863, 3) -> (16.7863, 0)
  line L494 (16.7863, 0) -> (31.7863, 0)
  line L495 (31.7863, 0) -> (31.7863, 3)
  line L496 (31.7863, 3) -> (43, 3)
  line L497 (43, 3) -> (43, 11.25)
  line L498 (43, 11.25) -> (40, 11.25)
  line L499 (40, 11.25) -> (40, 26.25)
  line L500 (40, 26.25) -> (43, 26.25)
  line L501 (43, 26.25) -> (43, 37.5)
  line L502 (43, 37.5) -> (40, 37.5)
  line L503 (40, 37.5) -> (40, 52.5)
  line L504 (40, 52.5) -> (43, 52.5)
  line L505 (43, 52.5) -> (43, 63.75)
  line L506 (43, 63.75) -> (40, 63.75)
  line L507 (40, 63.75) -> (40, 78.75)
  line L508 (40, 78.75) -> (43, 78.75)
  line L509 (43, 78.75) -> (43, 160)
  line L510 (43, 160) -> (-43, 160)
  line L511 (-43, 160) -> (-43, 78.75)
  line L512 (-43, 78.75) -> (-40, 78.75)
  line L513 (-40, 78.75) -> (-40, 63.75)
  line L514 (-40, 63.75) -> (-43, 63.75)
  line L515 (-43, 63.75) -> (-43, 52.5)
  line L516 (-43, 52.5) -> (-40, 52.5)
  line L517 (-40, 52.5) -> (-40, 37.5)
  line L518 (-40, 37.5) -> (-43, 37.5)
  line L519 (-43, 37.5) -> (-43, 26.25)
  line L520 (-43, 26.25) -> (-40, 26.25)
  line L521 (-40, 26.25) -> (-40, 11.25)
  line L522 (-40, 11.25) -> (-43, 11.25)
  line L523 (-43, 11.25) -> (-43, 3)
  line L524 (-19.4788, 143.8773) -> (17.7289, 143.8745) construction
  line L525 (17.7289, 143.8745) -> (17.7298, 155.0813) construction
  line L526 (17.7298, 155.0813) -> (-19.4779, 155.084) construction
  line L527 (-19.4779, 155.084) -> (-19.4788, 143.8773) construction
  dimension "d26" = 12
copy_body "Cuerpo - > Comp.1" bodies 2 removing the originals makes body 4 in component "Component"
fillet "Empalme1" radius 10 1 edges at (43, -38.5, 160) on bodies 4 in component "Component"
fillet "Empalme2" radius 10 1 edges at (-43, -38.5, 160) on bodies 4 in component "Component"
sketch "Boceto8" plane through (0, -37, 0) normal (0, 1, 0) x (-1, 0, 0)
copy_body "Cuerpo - > Comp.3" bodies 3 removing the originals makes body 5 in component "Component'"
copy_body "Cuerpo - > Comp.1'" bodies 4 removing the originals makes body 6 in component "Component''"
component "Component" placed x (1, 0, 0) y (0, 1, 0) z (0, 0, 1) at (0, 0, 0)
component "Component'" placed x (1, 0, 0) y (0, 1, 0) z (0, 0, 1) at (0, 0, 0)
component "Component'''" placed x (1, 0, 0) y (0, 1, 0) z (0, 0, 1) at (0, 0, 0)
component "Component''" placed x (1, 0, 0) y (0, 1, 0) z (0, 0, 1) at (0, 0, 0) in component "Component"
